Autodesk Inventor part; units mm, degrees
(part 2 of 3)
  line L262 (13.6018, -17.5742) -> (13.2961, -17.2686)
  spline S264 degree 2 poles (13.2961, -17.2686) (13.3171, -17.2092) (13.3852, -17.0328) (13.4219, -16.9716) knots 0 0 0 1 2 2 2
  spline S265 degree 2 poles (13.4219, -16.9716) (13.4708, -16.8808) (13.5599, -16.7498) (13.6454, -16.6642) knots 0 0 0 1 2 2 2
  spline S266 degree 2 poles (12.2779, -18.0318) (12.4455, -17.8641) (12.8263, -17.6895) (13.0306, -17.6947) knots 0 0 0 1 2 2 2
  spline S267 degree 2 poles (13.0306, -17.6947) (13.2332, -17.6982) (13.6612, -17.906) (13.8742, -18.1191) knots 0 0 0 1 2 2 2
  spline S268 degree 2 poles (13.8742, -18.1191) (14.0873, -18.3322) (14.2847, -18.7566) (14.2934, -18.9575) knots 0 0 0 1 2 2 2
  spline S269 degree 2 poles (14.2934, -18.9575) (14.3039, -19.1601) (14.1327, -19.5583) (13.9686, -19.7225) knots 0 0 0 1 2 2 2
  spline S270 degree 2 poles (13.9686, -19.7225) (13.8358, -19.8552) (13.5127, -20.0281) (13.3677, -20.0753) knots 0 0 0 1 2 2 2
  line L263 (13.3677, -20.0753) -> (13.0621, -19.7696)
  line L264 (13.0621, -19.7696) -> (13.0778, -19.7539)
  spline S271 degree 2 poles (13.0778, -19.7539) (13.1319, -19.7487) (13.2856, -19.7207) (13.3835, -19.6893) knots 0 0 0 1 2 2 2
  spline S272 degree 2 poles (13.3835, -19.6893) (13.469, -19.6596) (13.6664, -19.5496) (13.7363, -19.4797) knots 0 0 0 1 2 2 2
  spline S273 degree 2 poles (13.7363, -19.4797) (13.9476, -19.2684) (13.8847, -18.692) (13.593, -18.4003) knots 0 0 0 1 2 2 2
  spline S274 degree 2 poles (13.593, -18.4003) (13.3084, -18.1156) (12.7407, -18.044) (12.5207, -18.2641) knots 0 0 0 1 2 2 2
  spline S275 degree 2 poles (12.5207, -18.2641) (12.3879, -18.3968) (12.2569, -18.7479) (12.2499, -18.926) knots 0 0 0 1 2 2 2
  line L265 (12.2499, -18.926) -> (12.2342, -18.9418)
  line L266 (12.2342, -18.9418) -> (11.9286, -18.6361)
  spline S276 degree 2 poles (11.9286, -18.6361) (11.9495, -18.5767) (12.0176, -18.4003) (12.0543, -18.3392) knots 0 0 0 1 2 2 2
  spline S277 degree 2 poles (12.0543, -18.3392) (12.1032, -18.2484) (12.1923, -18.1174) (12.2779, -18.0318) knots 0 0 0 1 2 2 2
  line L267 (11.312, -19.071) -> (11.5845, -18.7985)
  line L268 (11.5845, -18.7985) -> (13.2018, -20.4159)
  line L269 (13.2018, -20.4159) -> (12.9293, -20.6883)
  line L270 (12.9293, -20.6883) -> (11.312, -19.071)
  line L271 (13.1791, -20.9765) -> (13.4882, -20.6674)
  line L272 (13.4882, -20.6674) -> (13.7712, -20.9503)
  line L273 (13.7712, -20.9503) -> (13.462, -21.2595)
  line L274 (13.462, -21.2595) -> (13.1791, -20.9765)
  spline S278 degree 2 poles (10.3916, -21.6088) (9.9829, -21.2001) (9.9305, -20.3617) (10.2588, -20.0334) knots 0 0 0 1 2 2 2
  spline S279 degree 2 poles (10.2588, -20.0334) (10.5959, -19.6963) (11.4413, -19.7696) (11.836, -20.1644) knots 0 0 0 1 2 2 2
  spline S280 degree 2 poles (11.836, -20.1644) (12.2412, -20.5696) (12.2919, -21.4166) (11.967, -21.7415) knots 0 0 0 1 2 2 2
  spline S281 degree 2 poles (11.967, -21.7415) (11.6386, -22.0699) (10.7985, -22.0157) (10.3916, -21.6088) knots 0 0 0 1 2 2 2
  spline S282 degree 2 poles (10.6728, -21.3276) (10.9872, -21.642) (11.5216, -21.7188) (11.7329, -21.5075) knots 0 0 0 1 2 2 2
  spline S283 degree 2 poles (11.7329, -21.5075) (11.9443, -21.2961) (11.8692, -20.7599) (11.5548, -20.4456) knots 0 0 0 1 2 2 2
  spline S284 degree 2 poles (11.5548, -20.4456) (11.2492, -20.1399) (10.7042, -20.0561) (10.4929, -20.2674) knots 0 0 0 1 2 2 2
  spline S285 degree 2 poles (10.4929, -20.2674) (10.2833, -20.477) (10.3619, -21.0167) (10.6728, -21.3276) knots 0 0 0 1 2 2 2
  line L275 (14.7087, -8.5772) -> (15.9575, -7.3284)
  line L276 (15.9575, -7.3284) -> (18.1127, -9.4837)
  line L277 (18.1127, -9.4837) -> (17.8263, -9.7701)
  line L278 (17.8263, -9.7701) -> (15.926, -7.8699)
  line L279 (15.926, -7.8699) -> (14.9637, -8.8322)
  line L280 (14.9637, -8.8322) -> (14.7087, -8.5772)
  spline S286 degree 2 poles (13.7655, -9.447) (14.1533, -9.0593) (15.0143, -9.068) (15.416, -9.4697) knots 0 0 0 1 2 2 2
  spline S287 degree 2 poles (15.416, -9.4697) (15.8107, -9.8644) (15.8649, -10.7464) (15.5313, -11.08) knots 0 0 0 1 2 2 2
  spline S288 degree 2 poles (15.5313, -11.08) (15.3811, -11.2302) (15.0615, -11.3752) (14.8833, -11.3682) knots 0 0 0 1 2 2 2
  spline S289 degree 2 poles (14.8833, -11.3682) (14.7034, -11.363) (14.3436, -11.1883) (14.1498, -10.9945) knots 0 0 0 1 2 2 2
  line L281 (14.1498, -10.9945) -> (14.0013, -10.846)
  line L282 (14.0013, -10.846) -> (15.1209, -9.7265)
  spline S290 degree 2 poles (15.1209, -9.7265) (14.8397, -9.4453) (14.258, -9.4295) (14.0065, -9.681) knots 0 0 0 1 2 2 2
  spline S291 degree 2 poles (14.0065, -9.681) (13.9175, -9.7701) (13.7847, -9.9832) (13.7463, -10.0845) knots 0 0 0 1 2 2 2
  spline S292 degree 2 poles (13.7463, -10.0845) (13.7079, -10.1928) (13.6677, -10.3552) (13.6625, -10.4163) knots 0 0 0 1 2 2 2
  line L283 (13.6625, -10.4163) -> (13.6468, -10.4321)
  line L284 (13.6468, -10.4321) -> (13.3498, -10.1351)
  spline S293 degree 2 poles (13.3498, -10.1351) (13.3778, -10.0688) (13.4651, -9.8697) (13.5053, -9.7981) knots 0 0 0 1 2 2 2
  spline S294 degree 2 poles (13.5053, -9.7981) (13.5612, -9.6968) (13.6677, -9.5448) (13.7655, -9.447) knots 0 0 0 1 2 2 2
  spline S295 degree 2 poles (14.4746, -10.7884) (14.5881, -10.8949) (14.7942, -11.0102) (14.8921, -11.0207) knots 0 0 0 1 2 2 2
  spline S296 degree 2 poles (14.8921, -11.0207) (15.0003, -11.0346) (15.2134, -10.9508) (15.3235, -10.8408) knots 0 0 0 1 2 2 2
  spline S297 degree 2 poles (15.3235, -10.8408) (15.4317, -10.7325) (15.5191, -10.5159) (15.5191, -10.3901) knots 0 0 0 1 2 2 2
  spline S298 degree 2 poles (15.5191, -10.3901) (15.5156, -10.2644) (15.423, -10.0461) (15.3287, -9.9343) knots 0 0 0 1 2 2 2
  line L285 (15.3287, -9.9343) -> (14.4746, -10.7884)
  spline S299 degree 2 poles (12.4242, -12.479) (12.0155, -12.0703) (11.9631, -11.232) (12.2914, -10.9036) knots 0 0 0 1 2 2 2
  spline S300 degree 2 poles (12.2914, -10.9036) (12.6285, -10.5665) (13.4738, -10.6399) (13.8686, -11.0346) knots 0 0 0 1 2 2 2
  spline S301 degree 2 poles (13.8686, -11.0346) (14.2738, -11.4398) (14.3244, -12.2869) (13.9996, -12.6118) knots 0 0 0 1 2 2 2
  spline S302 degree 2 poles (13.9996, -12.6118) (13.6712, -12.9401) (12.8311, -12.886) (12.4242, -12.479) knots 0 0 0 1 2 2 2
  spline S303 degree 2 poles (12.7054, -12.1978) (13.0197, -12.5122) (13.5542, -12.5891) (13.7655, -12.3777) knots 0 0 0 1 2 2 2
  spline S304 degree 2 poles (13.7655, -12.3777) (13.9769, -12.1664) (13.9017, -11.6302) (13.5874, -11.3158) knots 0 0 0 1 2 2 2
  spline S305 degree 2 poles (13.5874, -11.3158) (13.2817, -11.0102) (12.7368, -10.9263) (12.5255, -11.1377) knots 0 0 0 1 2 2 2
  spline S306 degree 2 poles (12.5255, -11.1377) (12.3159, -11.3473) (12.3945, -11.887) (12.7054, -12.1978) knots 0 0 0 1 2 2 2
  line L286 (10.0663, -13.2196) -> (10.3388, -12.9471)
  line L287 (10.3388, -12.9471) -> (11.2609, -13.8693)
  spline S307 degree 2 poles (11.2609, -13.8693) (11.3727, -13.9811) (11.5858, -14.1522) (11.6749, -14.1784) knots 0 0 0 1 2 2 2
  spline S308 degree 2 poles (11.6749, -14.1784) (11.7692, -14.2064) (11.9473, -14.147) (12.0486, -14.0457) knots 0 0 0 1 2 2 2
  spline S309 degree 2 poles (12.0486, -14.0457) (12.1499, -13.9444) (12.2565, -13.6213) (12.2722, -13.4309) knots 0 0 0 1 2 2 2
  line L288 (12.2722, -13.4309) -> (11.0636, -12.2223)
  line L289 (11.0636, -12.2223) -> (11.336, -11.9498)
  line L290 (11.336, -11.9498) -> (12.9534, -13.5671)
  line L291 (12.9534, -13.5671) -> (12.6809, -13.8396)
  line L292 (12.6809, -13.8396) -> (12.501, -13.6597)
  spline S310 degree 2 poles (12.501, -13.6597) (12.4888, -13.892) (12.3683, -14.2431) (12.2355, -14.3758) knots 0 0 0 1 2 2 2
  spline S311 degree 2 poles (12.2355, -14.3758) (11.998, -14.6133) (11.4146, -14.5679) (11.116, -14.2693) knots 0 0 0 1 2 2 2
  line L293 (11.116, -14.2693) -> (10.0663, -13.2196)
  spline S312 degree 2 poles (8.9537, -14.6745) (8.9625, -14.6168) (8.9869, -14.4177) (9.0131, -14.3391) knots 0 0 0 1 2 2 2
  spline S313 degree 2 poles (9.0131, -14.3391) (9.0463, -14.2291) (9.1406, -14.0544) (9.2629, -13.9322) knots 0 0 0 1 2 2 2
  spline S314 degree 2 poles (9.2629, -13.9322) (9.3624, -13.8326) (9.6174, -13.7278) (9.7537, -13.7278) knots 0 0 0 1 2 2 2
  spline S315 degree 2 poles (9.7537, -13.7278) (9.8846, -13.7296) (10.1589, -13.8466) (10.2671, -13.9549) knots 0 0 0 1 2 2 2
  spline S316 degree 2 poles (10.2671, -13.9549) (10.4348, -14.1226) (10.5309, -14.5016) (10.4453, -14.7234) knots 0 0 0 1 2 2 2
  spline S317 degree 2 poles (10.4453, -14.7234) (10.3719, -14.9225) (10.0488, -15.3399) (9.8462, -15.567) knots 0 0 0 1 2 2 2
  line L294 (9.8462, -15.567) -> (9.8986, -15.6194)
  spline S318 degree 2 poles (9.8986, -15.6194) (9.9929, -15.7137) (10.1676, -15.7731) (10.2532, -15.7538) knots 0 0 0 1 2 2 2
  spline S319 degree 2 poles (10.2532, -15.7538) (10.3388, -15.7346) (10.5099, -15.6054) (10.5903, -15.525) knots 0 0 0 1 2 2 2
  spline S320 degree 2 poles (10.5903, -15.525) (10.6846, -15.4307) (10.8837, -15.1198) (10.957, -14.9382) knots 0 0 0 1 2 2 2
  line L295 (10.957, -14.9382) -> (10.9728, -14.9225)
  line L296 (10.9728, -14.9225) -> (11.2505, -15.2002)
  spline S321 degree 2 poles (11.2505, -15.2002) (11.1963, -15.2962) (10.9675, -15.6298) (10.8295, -15.7678) knots 0 0 0 1 2 2 2
  spline S322 degree 2 poles (10.8295, -15.7678) (10.6619, -15.9355) (10.3807, -16.1119) (10.2217, -16.1346) knots 0 0 0 1 2 2 2
  spline S323 degree 2 poles (10.2217, -16.1346) (10.0663, -16.1573) (9.7676, -16.0333) (9.6157, -15.8813) knots 0 0 0 1 2 2 2
  line L297 (9.6157, -15.8813) -> (8.5101, -14.7758)
  line L298 (8.5101, -14.7758) -> (8.7826, -14.5033)
  line L299 (8.7826, -14.5033) -> (8.9537, -14.6745)
  line L300 (9.1808, -14.9015) -> (9.6297, -15.3504)
  spline S324 degree 2 poles (9.6297, -15.3504) (9.7187, -15.2439) (9.9842, -14.919) (10.0488, -14.7985) knots 0 0 0 1 2 2 2
  spline S325 degree 2 poles (10.0488, -14.7985) (10.1239, -14.657) (10.1274, -14.3776) (10.0052, -14.2553) knots 0 0 0 1 2 2 2
  spline S326 degree 2 poles (10.0052, -14.2553) (9.8654, -14.1156) (9.5668, -14.1313) (9.4166, -14.2815) knots 0 0 0 1 2 2 2
  spline S327 degree 2 poles (9.4166, -14.2815) (9.2891, -14.409) (9.1895, -14.7286) (9.1808, -14.9015) knots 0 0 0 1 2 2 2
  line L301 (8.5957, -17.3415) -> (8.6097, -17.3275)
  spline S328 degree 2 poles (8.6097, -17.3275) (8.6498, -17.3048) (8.7214, -17.2402) (8.7686, -17.193) knots 0 0 0 1 2 2 2
  spline S329 degree 2 poles (8.7686, -17.193) (8.8786, -17.083) (8.9991, -16.7703) (9.0026, -16.5782) knots 0 0 0 1 2 2 2
  line L302 (9.0026, -16.5782) -> (7.8551, -15.4307)
  line L303 (7.8551, -15.4307) -> (8.1276, -15.1583)
  line L304 (8.1276, -15.1583) -> (9.7449, -16.7756)
  line L305 (9.7449, -16.7756) -> (9.4725, -17.0481)
  line L306 (9.4725, -17.0481) -> (9.2314, -16.807)
  spline S330 degree 2 poles (9.2314, -16.807) (9.2157, -17.0882) (9.1022, -17.4183) (8.9974, -17.5231) knots 0 0 0 1 2 2 2
  spline S331 degree 2 poles (8.9974, -17.5231) (8.9555, -17.565) (8.9101, -17.6035) (8.8786, -17.6244) knots 0 0 0 1 2 2 2
  line L307 (8.8786, -17.6244) -> (8.5957, -17.3415)
  line L308 (5.8152, -17.4707) -> (6.0876, -17.1983)
  line L309 (6.0876, -17.1983) -> (6.2518, -17.3624)
  spline S332 degree 2 poles (6.2518, -17.3624) (6.2623, -17.2472) (6.285, -17.0847) (6.3182, -16.9922) knots 0 0 0 1 2 2 2
  spline S333 degree 2 poles (6.3182, -16.9922) (6.3479, -16.9066) (6.4422, -16.7529) (6.5243, -16.6708) knots 0 0 0 1 2 2 2
  spline S334 degree 2 poles (6.5243, -16.6708) (6.657, -16.5381) (6.9906, -16.4245) (7.1757, -16.4525) knots 0 0 0 1 2 2 2
  spline S335 degree 2 poles (7.1757, -16.4525) (7.3609, -16.4804) (7.7626, -16.7075) (7.9669, -16.9118) knots 0 0 0 1 2 2 2
  spline S336 degree 2 poles (7.9669, -16.9118) (8.18, -17.1249) (8.3809, -17.5458) (8.4018, -17.7589) knots 0 0 0 1 2 2 2
  spline S337 degree 2 poles (8.4018, -17.7589) (8.4175, -17.9528) (8.2883, -18.323) (8.1503, -18.461) knots 0 0 0 1 2 2 2
  spline S338 degree 2 poles (8.1503, -18.461) (8.0298, -18.5815) (7.7958, -18.7073) (7.6403, -18.751) knots 0 0 0 1 2 2 2
  line L310 (7.6403, -18.751) -> (8.3389, -19.4496)
  line L311 (8.3389, -19.4496) -> (8.0665, -19.722)
  line L312 (8.0665, -19.722) -> (5.8152, -17.4707)
  line L313 (6.4806, -17.5912) -> (7.415, -18.5256)
  spline S339 degree 2 poles (7.415, -18.5256) (7.5652, -18.4732) (7.7626, -18.3492) (7.8551, -18.2567) knots 0 0 0 1 2 2 2
  spline S340 degree 2 poles (7.8551, -18.2567) (8.0647, -18.0471) (7.9879, -17.4952) (7.691, -17.1983) knots 0 0 0 1 2 2 2
  spline S341 degree 2 poles (7.691, -17.1983) (7.4045, -16.9118) (6.9207, -16.7913) (6.7199, -16.9922) knots 0 0 0 1 2 2 2
  spline S342 degree 2 poles (6.7199, -16.9922) (6.6133, -17.0987) (6.4946, -17.4131) (6.4806, -17.5912) knots 0 0 0 1 2 2 2
  spline S343 degree 2 poles (4.9, -20.0032) (4.4913, -19.5945) (4.4389, -18.7562) (4.7672, -18.4278) knots 0 0 0 1 2 2 2
  spline S344 degree 2 poles (4.7672, -18.4278) (5.1043, -18.0908) (5.9496, -18.1641) (6.3444, -18.5588) knots 0 0 0 1 2 2 2
  spline S345 degree 2 poles (6.3444, -18.5588) (6.7496, -18.964) (6.8002, -19.8111) (6.4754, -20.136) knots 0 0 0 1 2 2 2
  spline S346 degree 2 poles (6.4754, -20.136) (6.147, -20.4643) (5.3069, -20.4102) (4.9, -20.0032) knots 0 0 0 1 2 2 2
  spline S347 degree 2 poles (5.1811, -19.722) (5.4955, -20.0364) (6.03, -20.1133) (6.2413, -19.9019) knots 0 0 0 1 2 2 2
  spline S348 degree 2 poles (6.2413, -19.9019) (6.4526, -19.6906) (6.3775, -19.1544) (6.0632, -18.84) knots 0 0 0 1 2 2 2
  spline S349 degree 2 poles (6.0632, -18.84) (5.7575, -18.5344) (5.2126, -18.4505) (5.0013, -18.6619) knots 0 0 0 1 2 2 2
  spline S350 degree 2 poles (5.0013, -18.6619) (4.7917, -18.8715) (4.8703, -19.4112) (5.1811, -19.722) knots 0 0 0 1 2 2 2
  line L314 (-17.3745, -18.836) -> (-14.477, -17.4231)
  line L315 (-14.477, -17.4231) -> (-14.1679, -17.7322)
  line L316 (-14.1679, -17.7322) -> (-15.5808, -20.6297)
  line L317 (-15.5808, -20.6297) -> (-15.8882, -20.3224)
  line L318 (-15.8882, -20.3224) -> (-14.6953, -17.9348)
  line L319 (-14.6953, -17.9348) -> (-17.0829, -19.1277)
  line L320 (-17.0829, -19.1277) -> (-17.3745, -18.836)
  line L321 (-15.6821, -16.2179) -> (-15.4097, -16.4904)
  line L322 (-15.4097, -16.4904) -> (-17.027, -18.1077)
  line L323 (-17.027, -18.1077) -> (-17.2994, -17.8352)
  line L324 (-17.2994, -17.8352) -> (-15.6821, -16.2179)
  line L325 (-17.5876, -18.085) -> (-17.2785, -18.3941)
  line L326 (-17.2785, -18.3941) -> (-17.5614, -18.6771)
  line L327 (-17.5614, -18.6771) -> (-17.8706, -18.3679)
  line L328 (-17.8706, -18.3679) -> (-17.5876, -18.085)
  spline S351 degree 2 poles (-16.5397, -15.2975) (-16.3179, -15.5193) (-16.3214, -16.0223) (-16.5956, -16.2965) knots 0 0 0 1 2 2 2
  line L329 (-16.5956, -16.2965) -> (-17.4916, -17.1925)
  line L330 (-17.4916, -17.1925) -> (-17.3082, -17.3759)
  line L331 (-17.3082, -17.3759) -> (-17.5335, -17.6012)
  line L332 (-17.5335, -17.6012) -> (-17.7169, -17.4178)
  line L333 (-17.7169, -17.4178) -> (-18.1815, -17.8824)
  line L334 (-18.1815, -17.8824) -> (-18.4539, -17.6099)
  line L335 (-18.4539, -17.6099) -> (-17.9893, -17.1454)
  line L336 (-17.9893, -17.1454) -> (-18.4906, -16.6441)
  line L337 (-18.4906, -16.6441) -> (-18.2653, -16.4188)
  line L338 (-18.2653, -16.4188) -> (-17.764, -16.92)
  line L339 (-17.764, -16.92) -> (-16.9938, -16.1498)
  spline S352 degree 2 poles (-16.9938, -16.1498) (-16.8715, -16.0275) (-16.7458, -15.8843) (-16.7178, -15.797) knots 0 0 0 1 2 2 2
  spline S353 degree 2 poles (-16.7178, -15.797) (-16.6916, -15.7219) (-16.751, -15.5612) (-16.8453, -15.4669) knots 0 0 0 1 2 2 2
  spline S354 degree 2 poles (-16.8453, -15.4669) (-16.9117, -15.4005) (-17.0759, -15.3167) (-17.1161, -15.301) knots 0 0 0 1 2 2 2
  line L340 (-17.1161, -15.301) -> (-17.1318, -15.2853)
  line L341 (-17.1318, -15.2853) -> (-16.8873, -15.0407)
  spline S355 degree 2 poles (-16.8873, -15.0407) (-16.7894, -15.0966) (-16.6078, -15.2294) (-16.5397, -15.2975) knots 0 0 0 1 2 2 2
  spline S356 degree 2 poles (-17.5317, -14.3054) (-17.3099, -14.5272) (-17.3134, -15.0303) (-17.5876, -15.3045) knots 0 0 0 1 2 2 2
  line L342 (-17.5876, -15.3045) -> (-18.4836, -16.2005)
  line L343 (-18.4836, -16.2005) -> (-18.3002, -16.3838)
  line L344 (-18.3002, -16.3838) -> (-18.5255, -16.6092)
  line L345 (-18.5255, -16.6092) -> (-18.7089, -16.4258)
  line L346 (-18.7089, -16.4258) -> (-19.1735, -16.8904)
  line L347 (-19.1735, -16.8904) -> (-19.446, -16.6179)
  line L348 (-19.446, -16.6179) -> (-18.9814, -16.1533)
  line L349 (-18.9814, -16.1533) -> (-19.4827, -15.652)
  line L350 (-19.4827, -15.652) -> (-19.2573, -15.4267)
  line L351 (-19.2573, -15.4267) -> (-18.7561, -15.928)
  line L352 (-18.7561, -15.928) -> (-17.9858, -15.1578)
  spline S357 degree 2 poles (-17.9858, -15.1578) (-17.8636, -15.0355) (-17.7378, -14.8923) (-17.7099, -14.805) knots 0 0 0 1 2 2 2
  spline S358 degree 2 poles (-17.7099, -14.805) (-17.6837, -14.7299) (-17.7431, -14.5692) (-17.8374, -14.4749) knots 0 0 0 1 2 2 2
  spline S359 degree 2 poles (-17.8374, -14.4749) (-17.9038, -14.4085) (-18.0679, -14.3246) (-18.1081, -14.3089) knots 0 0 0 1 2 2 2
  line L353 (-18.1081, -14.3089) -> (-18.1238, -14.2932)
  line L354 (-18.1238, -14.2932) -> (-17.8793, -14.0487)
  spline S360 degree 2 poles (-17.8793, -14.0487) (-17.7815, -14.1046) (-17.5999, -14.2373) (-17.5317, -14.3054) knots 0 0 0 1 2 2 2
  line L355 (-18.3439, -13.5562) -> (-18.0714, -13.8286)
  line L356 (-18.0714, -13.8286) -> (-19.6887, -15.4459)
  line L357 (-19.6887, -15.4459) -> (-19.9612, -15.1735)
  line L358 (-19.9612, -15.1735) -> (-18.3439, -13.5562)
  line L359 (-20.2494, -15.4232) -> (-19.9403, -15.7324)
  line L360 (-19.9403, -15.7324) -> (-20.2232, -16.0153)
  line L361 (-20.2232, -16.0153) -> (-20.5323, -15.7062)
  line L362 (-20.5323, -15.7062) -> (-20.2494, -15.4232)
  spline S361 degree 2 poles (-8.1645, -16.5546) (-7.9357, -16.7834) (-7.6964, -17.3021) (-7.7016, -17.5798) knots 0 0 0 1 2 2 2
  spline S362 degree 2 poles (-7.7016, -17.5798) (-7.7086, -17.8593) (-7.9863, -18.4269) (-8.2605, -18.7011) knots 0 0 0 1 2 2 2
  spline S363 degree 2 poles (-8.2605, -18.7011) (-8.5208, -18.9613) (-9.0797, -19.2268) (-9.3626, -19.2373) knots 0 0 0 1 2 2 2
  spline S364 degree 2 poles (-9.3626, -19.2373) (-9.6351, -19.2478) (-10.173, -19.0172) (-10.4018, -18.7884) knots 0 0 0 1 2 2 2
  spline S365 degree 2 poles (-10.4018, -18.7884) (-10.5119, -18.6784) (-10.6795, -18.4479) (-10.7424, -18.3291) knots 0 0 0 1 2 2 2
  spline S366 degree 2 poles (-10.7424, -18.3291) (-10.7948, -18.2348) (-10.8961, -17.9798) (-10.9223, -17.8977) knots 0 0 0 1 2 2 2
  line L363 (-10.9223, -17.8977) -> (-10.5765, -17.5519)
  line L364 (-10.5765, -17.5519) -> (-10.552, -17.5763)
  spline S367 degree 2 poles (-10.552, -17.5763) (-10.545, -17.6776) (-10.5171, -17.8767) (-10.4612, -18.0304) knots 0 0 0 1 2 2 2
  spline S368 degree 2 poles (-10.4612, -18.0304) (-10.4175, -18.1614) (-10.2499, -18.4444) (-10.1206, -18.5736) knots 0 0 0 1 2 2 2
  spline S369 degree 2 poles (-10.1206, -18.5736) (-9.8097, -18.8845) (-8.9574, -18.8007) (-8.5679, -18.4112) knots 0 0 0 1 2 2 2
  spline S370 degree 2 poles (-8.5679, -18.4112) (-8.3514, -18.1946) (-8.1278, -17.7684) (-8.1121, -17.5606) knots 0 0 0 1 2 2 2
  spline S371 degree 2 poles (-8.1121, -17.5606) (-8.0929, -17.3563) (-8.2378, -16.9772) (-8.402, -16.8131) knots 0 0 0 1 2 2 2
  spline S372 degree 2 poles (-8.402, -16.8131) (-8.5225, -16.6926) (-8.7985, -16.4865) (-8.9155, -16.4393) knots 0 0 0 1 2 2 2
  line L365 (-8.9155, -16.4393) -> (-9.4727, -16.9965)
  line L366 (-9.4727, -16.9965) -> (-8.9731, -17.496)
  line L367 (-8.9731, -17.496) -> (-9.2246, -17.7475)
  line L368 (-9.2246, -17.7475) -> (-10.0071, -16.965)
  line L369 (-10.0071, -16.965) -> (-9.0657, -16.0236)
  spline S373 degree 2 poles (-9.0657, -16.0236) (-8.9871, -16.0533) (-8.7269, -16.1633) (-8.6256, -16.2192) knots 0 0 0 1 2 2 2
  spline S374 degree 2 poles (-8.6256, -16.2192) (-8.4876, -16.2943) (-8.285, -16.4341) (-8.1645, -16.5546) knots 0 0 0 1 2 2 2
  spline S375 degree 2 poles (-10.3337, -14.8115) (-10.2761, -14.8202) (-10.077, -14.8447) (-9.9984, -14.8709) knots 0 0 0 1 2 2 2
  spline S376 degree 2 poles (-9.9984, -14.8709) (-9.8883, -14.9041) (-9.7137, -14.9984) (-9.5914, -15.1206) knots 0 0 0 1 2 2 2
  spline S377 degree 2 poles (-9.5914, -15.1206) (-9.4919, -15.2202) (-9.3871, -15.4752) (-9.3871, -15.6114) knots 0 0 0 1 2 2 2
  spline S378 degree 2 poles (-9.3871, -15.6114) (-9.3888, -15.7424) (-9.5058, -16.0166) (-9.6141, -16.1249) knots 0 0 0 1 2 2 2
  spline S379 degree 2 poles (-9.6141, -16.1249) (-9.7818, -16.2926) (-10.1608, -16.3887) (-10.3826, -16.3031) knots 0 0 0 1 2 2 2
  spline S380 degree 2 poles (-10.3826, -16.3031) (-10.5817, -16.2297) (-10.9992, -15.9066) (-11.2262, -15.704) knots 0 0 0 1 2 2 2
  line L370 (-11.2262, -15.704) -> (-11.2786, -15.7564)
  spline S381 degree 2 poles (-11.2786, -15.7564) (-11.3729, -15.8507) (-11.4323, -16.0254) (-11.4131, -16.111) knots 0 0 0 1 2 2 2
  spline S382 degree 2 poles (-11.4131, -16.111) (-11.3939, -16.1965) (-11.2646, -16.3677) (-11.1843, -16.448) knots 0 0 0 1 2 2 2
  spline S383 degree 2 poles (-11.1843, -16.448) (-11.09, -16.5424) (-10.7791, -16.7415) (-10.5974, -16.8148) knots 0 0 0 1 2 2 2
  line L371 (-10.5974, -16.8148) -> (-10.5817, -16.8305)
  line L372 (-10.5817, -16.8305) -> (-10.8594, -17.1082)
  spline S384 degree 2 poles (-10.8594, -17.1082) (-10.9555, -17.0541) (-11.2891, -16.8253) (-11.4271, -16.6873) knots 0 0 0 1 2 2 2
  spline S385 degree 2 poles (-11.4271, -16.6873) (-11.5947, -16.5196) (-11.7711, -16.2384) (-11.7938, -16.0795) knots 0 0 0 1 2 2 2
  spline S386 degree 2 poles (-11.7938, -16.0795) (-11.8165, -15.9241) (-11.6925, -15.6254) (-11.5406, -15.4735) knots 0 0 0 1 2 2 2
  line L373 (-11.5406, -15.4735) -> (-10.435, -14.3679)
  line L374 (-10.435, -14.3679) -> (-10.1625, -14.6403)
  line L375 (-10.1625, -14.6403) -> (-10.3337, -14.8115)
  line L376 (-10.5608, -15.0386) -> (-11.0096, -15.4874)
  spline S387 degree 2 poles (-11.0096, -15.4874) (-10.9031, -15.5765) (-10.5782, -15.842) (-10.4577, -15.9066) knots 0 0 0 1 2 2 2
  spline S388 degree 2 poles (-10.4577, -15.9066) (-10.3162, -15.9817) (-10.0368, -15.9852) (-9.9145, -15.8629) knots 0 0 0 1 2 2 2
  spline S389 degree 2 poles (-9.9145, -15.8629) (-9.7748, -15.7232) (-9.7905, -15.4246) (-9.9407, -15.2743) knots 0 0 0 1 2 2 2
  spline S390 degree 2 poles (-9.9407, -15.2743) (-10.0682, -15.1468) (-10.3879, -15.0473) (-10.5608, -15.0386) knots 0 0 0 1 2 2 2
  spline S391 degree 2 poles (-13.0077, -13.4649) (-12.6112, -13.0684) (-11.7432, -12.9689) (-11.4533, -13.2588) knots 0 0 0 1 2 2 2
  spline S392 degree 2 poles (-11.4533, -13.2588) (-11.3223, -13.3898) (-11.2, -13.6413) (-11.1651, -13.788) knots 0 0 0 1 2 2 2
  line L377 (-11.1651, -13.788) -> (-11.0725, -13.7304)
  line L378 (-11.0725, -13.7304) -> (-10.8175, -13.9854)
  line L379 (-10.8175, -13.9854) -> (-13.0688, -16.2367)
  line L380 (-13.0688, -16.2367) -> (-13.3413, -15.9642)
  line L381 (-13.3413, -15.9642) -> (-12.5379, -15.1608)
  spline S393 degree 2 poles (-12.5379, -15.1608) (-12.7335, -15.1503) (-13.095, -15.0333) (-13.247, -14.8814) knots 0 0 0 1 2 2 2
  spline S394 degree 2 poles (-13.247, -14.8814) (-13.5212, -14.6072) (-13.3972, -13.8544) (-13.0077, -13.4649) knots 0 0 0 1 2 2 2
  spline S395 degree 2 poles (-12.7055, -13.7251) (-12.9955, -14.0151) (-13.1195, -14.4919) (-12.9239, -14.6875) knots 0 0 0 1 2 2 2
  spline S396 degree 2 poles (-12.9239, -14.6875) (-12.8138, -14.7975) (-12.482, -14.9198) (-12.3091, -14.932) knots 0 0 0 1 2 2 2
  line L382 (-12.3091, -14.932) -> (-11.3816, -14.0046)
  spline S397 degree 2 poles (-11.3816, -14.0046) (-11.434, -13.8509) (-11.5511, -13.65) (-11.6454, -13.5557) knots 0 0 0 1 2 2 2
  spline S398 degree 2 poles (-11.6454, -13.5557) (-11.8532, -13.3479) (-12.3859, -13.4055) (-12.7055, -13.7251) knots 0 0 0 1 2 2 2
  line L383 (-14.639, -12.8152) -> (-14.625, -12.8292)
  spline S399 degree 2 poles (-14.625, -12.8292) (-14.6023, -12.8693) (-14.5377, -12.9409) (-14.4905, -12.9881) knots 0 0 0 1 2 2 2
  spline S400 degree 2 poles (-14.4905, -12.9881) (-14.3805, -13.0981) (-14.0679, -13.2186) (-13.8757, -13.2221) knots 0 0 0 1 2 2 2
  line L384 (-13.8757, -13.2221) -> (-12.7283, -12.0746)
  line L385 (-12.7283, -12.0746) -> (-12.4558, -12.3471)
  line L386 (-12.4558, -12.3471) -> (-14.0731, -13.9644)
  line L387 (-14.0731, -13.9644) -> (-14.3456, -13.692)
  line L388 (-14.3456, -13.692) -> (-14.1045, -13.4509)
  spline S401 degree 2 poles (-14.1045, -13.4509) (-14.3857, -13.4352) (-14.7158, -13.3217) (-14.8206, -13.2169) knots 0 0 0 1 2 2 2
  spline S402 degree 2 poles (-14.8206, -13.2169) (-14.8626, -13.175) (-14.901, -13.1296) (-14.9219, -13.0981) knots 0 0 0 1 2 2 2
  line L389 (-14.9219, -13.0981) -> (-14.639, -12.8152)
  line L390 (-13.8024, -11.0005) -> (-13.5299, -11.273)
  line L391 (-13.5299, -11.273) -> (-15.1472, -12.8903)
  line L392 (-15.1472, -12.8903) -> (-15.4197, -12.6178)
  line L393 (-15.4197, -12.6178) -> (-13.8024, -11.0005)
  line L394 (-15.7079, -12.8676) -> (-15.3987, -13.1767)
  line L395 (-15.3987, -13.1767) -> (-15.6817, -13.4597)
  line L396 (-15.6817, -13.4597) -> (-15.9908, -13.1505)
  line L397 (-15.9908, -13.1505) -> (-15.7079, -12.8676)
  spline S403 degree 2 poles (-14.8678, -9.8617) (-14.4801, -10.2495) (-14.4888, -11.1105) (-14.8905, -11.5122) knots 0 0 0 1 2 2 2
  spline S404 degree 2 poles (-14.8905, -11.5122) (-15.2852, -11.907) (-16.1672, -11.9611) (-16.5008, -11.6275) knots 0 0 0 1 2 2 2
  spline S405 degree 2 poles (-16.5008, -11.6275) (-16.651, -11.4773) (-16.796, -11.1577) (-16.789, -10.9795) knots 0 0 0 1 2 2 2
  spline S406 degree 2 poles (-16.789, -10.9795) (-16.7838, -10.7996) (-16.6091, -10.4399) (-16.4152, -10.246) knots 0 0 0 1 2 2 2
  line L398 (-16.4152, -10.246) -> (-16.2668, -10.0975)
  line L399 (-16.2668, -10.0975) -> (-15.1472, -11.2171)
  spline S407 degree 2 poles (-15.1472, -11.2171) (-14.866, -10.9359) (-14.8503, -10.3543) (-15.1018, -10.1028) knots 0 0 0 1 2 2 2
  spline S408 degree 2 poles (-15.1018, -10.1028) (-15.1909, -10.0137) (-15.404, -9.881) (-15.5053, -9.8425) knots 0 0 0 1 2 2 2
  spline S409 degree 2 poles (-15.5053, -9.8425) (-15.6136, -9.8041) (-15.776, -9.7639) (-15.8371, -9.7587) knots 0 0 0 1 2 2 2
  line L400 (-15.8371, -9.7587) -> (-15.8529, -9.743)
  line L401 (-15.8529, -9.743) -> (-15.5559, -9.4461)
  spline S410 degree 2 poles (-15.5559, -9.4461) (-15.4896, -9.474) (-15.2905, -9.5613) (-15.2189, -9.6015) knots 0 0 0 1 2 2 2
  spline S411 degree 2 poles (-15.2189, -9.6015) (-15.1176, -9.6574) (-14.9656, -9.7639) (-14.8678, -9.8617) knots 0 0 0 1 2 2 2
  spline S412 degree 2 poles (-16.2092, -10.5708) (-16.3157, -10.6844) (-16.431, -10.8905) (-16.4414, -10.9883) knots 0 0 0 1 2 2 2
  spline S413 degree 2 poles (-16.4414, -10.9883) (-16.4554, -11.0966) (-16.3716, -11.3096) (-16.2616, -11.4197) knots 0 0 0 1 2 2 2
  spline S414 degree 2 poles (-16.2616, -11.4197) (-16.1533, -11.528) (-15.9367, -11.6153) (-15.8109, -11.6153) knots 0 0 0 1 2 2 2
  spline S415 degree 2 poles (-15.8109, -11.6153) (-15.6852, -11.6118) (-15.4669, -11.5192) (-15.3551, -11.4249) knots 0 0 0 1 2 2 2
  line L402 (-15.3551, -11.4249) -> (-16.2092, -10.5708)
  line L403 (-16.0397, -8.7632) -> (-15.7673, -9.0356)
  line L404 (-15.7673, -9.0356) -> (-18.0186, -11.2869)
  line L405 (-18.0186, -11.2869) -> (-18.2911, -11.0145)
  line L406 (-18.2911, -11.0145) -> (-16.0397, -8.7632)
  spline S416 degree 2 poles (-17.1051, -7.6244) (-16.7174, -8.0121) (-16.7261, -8.8732) (-17.1278, -9.2749) knots 0 0 0 1 2 2 2
  spline S417 degree 2 poles (-17.1278, -9.2749) (-17.5226, -9.6696) (-18.4046, -9.7238) (-18.7382, -9.3902) knots 0 0 0 1 2 2 2
  spline S418 degree 2 poles (-18.7382, -9.3902) (-18.8884, -9.24) (-19.0334, -8.9203) (-19.0264, -8.7422) knots 0 0 0 1 2 2 2
  spline S419 degree 2 poles (-19.0264, -8.7422) (-19.0211, -8.5623) (-18.8465, -8.2025) (-18.6526, -8.0086) knots 0 0 0 1 2 2 2
  line L407 (-18.6526, -8.0086) -> (-18.5041, -7.8602)
  line L408 (-18.5041, -7.8602) -> (-17.3846, -8.9797)
  spline S420 degree 2 poles (-17.3846, -8.9797) (-17.1034, -8.6985) (-17.0877, -8.1169) (-17.3392, -7.8654) knots 0 0 0 1 2 2 2
  spline S421 degree 2 poles (-17.3392, -7.8654) (-17.4283, -7.7763) (-17.6413, -7.6436) (-17.7426, -7.6052) knots 0 0 0 1 2 2 2
  spline S422 degree 2 poles (-17.7426, -7.6052) (-17.8509, -7.5668) (-18.0134, -7.5266) (-18.0745, -7.5213) knots 0 0 0 1 2 2 2
  line L409 (-18.0745, -7.5213) -> (-18.0902, -7.5056)
  line L410 (-18.0902, -7.5056) -> (-17.7933, -7.2087)
  spline S423 degree 2 poles (-17.7933, -7.2087) (-17.7269, -7.2367) (-17.5278, -7.324) (-17.4562, -7.3642) knots 0 0 0 1 2 2 2
  spline S424 degree 2 poles (-17.4562, -7.3642) (-17.3549, -7.42) (-17.203, -7.5266) (-17.1051, -7.6244) knots 0 0 0 1 2 2 2
  spline S425 degree 2 poles (-18.4465, -8.3335) (-18.553, -8.447) (-18.6683, -8.6531) (-18.6788, -8.7509) knots 0 0 0 1 2 2 2
  spline S426 degree 2 poles (-18.6788, -8.7509) (-18.6928, -8.8592) (-18.6089, -9.0723) (-18.4989, -9.1823) knots 0 0 0 1 2 2 2
  spline S427 degree 2 poles (-18.4989, -9.1823) (-18.3906, -9.2906) (-18.174, -9.3779) (-18.0483, -9.3779) knots 0 0 0 1 2 2 2
  spline S428 degree 2 poles (-18.0483, -9.3779) (-17.9225, -9.3744) (-17.7042, -9.2819) (-17.5924, -9.1876) knots 0 0 0 1 2 2 2
  line L411 (-17.5924, -9.1876) -> (-18.4465, -8.3335)
  dimension "d28" = 45
  dimension "d29" = 45
  dimension "d30" = 135
  dimension "d31" = 135
  constraints: 16 end point, 4 equal length, 4 horizontal, 8 other
  measures "d28" angle of L16 L17
  measures "d29" angle of L19 L18
  measures "d30" angle of L21 L20
  measures "d31" angle of L22 L23
extrude "Estrusione2" cut sketch "Schizzo4" against normal blind 1
sketch "Schizzo5" plane through (0, 10, 0) normal (0, 1, 0) x (1, 0, 0)
  line L0 (-18.4465, -8.3335) -> (-17.5924, -9.1876) projected
  line L1 (-17.7933, -7.2087) -> (-18.0902, -7.5056) projected
  line L2 (-18.0902, -7.5056) -> (-18.0745, -7.5213) projected
  line L3 (-17.3846, -8.9797) -> (-18.5041, -7.8602) projected
  line L4 (-18.5041, -7.8602) -> (-18.6526, -8.0086) projected
  line L5 (-15.7079, -12.8676) -> (-15.9908, -13.1505) projected
  line L6 (-15.9908, -13.1505) -> (-15.6817, -13.4597) projected
  line L7 (-15.6817, -13.4597) -> (-15.3987, -13.1767) projected
  line L8 (-15.3987, -13.1767) -> (-15.7079, -12.8676) projected
  line L9 (-14.639, -12.8152) -> (-14.9219, -13.0981) projected
  line L10 (-14.1045, -13.4509) -> (-14.3456, -13.692) projected
  line L11 (-14.3456, -13.692) -> (-14.0731, -13.9644) projected
  line L12 (-14.0731, -13.9644) -> (-12.4558, -12.3471) projected
  line L13 (-12.4558, -12.3471) -> (-12.7283, -12.0746) projected
  line L14 (-12.7283, -12.0746) -> (-13.8757, -13.2221) projected
  line L15 (-14.625, -12.8292) -> (-14.639, -12.8152) projected
  line L16 (-11.3816, -14.0046) -> (-12.3091, -14.932) projected
  line L17 (-12.5379, -15.1608) -> (-13.3413, -15.9642) projected
  line L18 (-13.3413, -15.9642) -> (-13.0688, -16.2367) projected
  line L19 (-13.0688, -16.2367) -> (-10.8175, -13.9854) projected
  line L20 (-10.8175, -13.9854) -> (-11.0725, -13.7304) projected
  line L21 (-11.0725, -13.7304) -> (-11.1651, -13.788) projected
  line L22 (-11.0096, -15.4874) -> (-10.5608, -15.0386) projected
  line L23 (-10.3337, -14.8115) -> (-10.1625, -14.6403) projected
  line L24 (-10.1625, -14.6403) -> (-10.435, -14.3679) projected
  line L25 (-10.435, -14.3679) -> (-11.5406, -15.4735) projected
  line L26 (-10.8594, -17.1082) -> (-10.5817, -16.8305) projected
  line L27 (-10.5817, -16.8305) -> (-10.5974, -16.8148) projected
  line L28 (-11.2786, -15.7564) -> (-11.2262, -15.704) projected
  line L29 (-20.2494, -15.4232) -> (-20.5323, -15.7062) projected
  line L30 (-20.5323, -15.7062) -> (-20.2232, -16.0153) projected
  line L31 (-20.2232, -16.0153) -> (-19.9403, -15.7324) projected
  line L32 (-19.9403, -15.7324) -> (-20.2494, -15.4232) projected
  line L33 (-17.8793, -14.0487) -> (-18.1238, -14.2932) projected
  line L34 (-18.1238, -14.2932) -> (-18.1081, -14.3089) projected
  line L35 (-17.9858, -15.1578) -> (-18.7561, -15.928) projected
  line L36 (-18.7561, -15.928) -> (-19.2573, -15.4267) projected
  line L37 (-19.2573, -15.4267) -> (-19.4827, -15.652) projected
  line L38 (-19.4827, -15.652) -> (-18.9814, -16.1533) projected
  line L39 (-18.9814, -16.1533) -> (-19.446, -16.6179) projected
  line L40 (-19.446, -16.6179) -> (-19.1735, -16.8904) projected
  line L41 (-19.1735, -16.8904) -> (-18.7089, -16.4258) projected
  line L42 (-18.7089, -16.4258) -> (-18.5255, -16.6092) projected
  line L43 (-18.5255, -16.6092) -> (-18.3002, -16.3838) projected
  line L44 (-18.3002, -16.3838) -> (-18.4836, -16.2005) projected
  line L45 (-18.4836, -16.2005) -> (-17.5876, -15.3045) projected
  line L46 (-17.5876, -18.085) -> (-17.8706, -18.3679) projected
  line L47 (-17.8706, -18.3679) -> (-17.5614, -18.6771) projected
  line L48 (-17.5614, -18.6771) -> (-17.2785, -18.3941) projected
  line L49 (-17.2785, -18.3941) -> (-17.5876, -18.085) projected
  line L50 (-17.3745, -18.836) -> (-17.0829, -19.1277) projected
  line L51 (-17.0829, -19.1277) -> (-14.6953, -17.9348) projected
  line L52 (-14.6953, -17.9348) -> (-15.8882, -20.3224) projected
  line L53 (-15.8882, -20.3224) -> (-15.5808, -20.6297) projected
  line L54 (-15.5808, -20.6297) -> (-14.1679, -17.7322) projected
  line L55 (-14.1679, -17.7322) -> (-14.477, -17.4231) projected
  line L56 (-14.477, -17.4231) -> (-17.3745, -18.836) projected
  line L57 (7.415, -18.5256) -> (6.4806, -17.5912) projected
  line L58 (5.8152, -17.4707) -> (8.0665, -19.722) projected
  line L59 (8.0665, -19.722) -> (8.3389, -19.4496) projected
  line L60 (8.3389, -19.4496) -> (7.6403, -18.751) projected
  line L61 (6.2518, -17.3624) -> (6.0876, -17.1983) projected
  line L62 (6.0876, -17.1983) -> (5.8152, -17.4707) projected
  line L63 (10.0663, -13.2196) -> (11.116, -14.2693) projected
  line L64 (12.501, -13.6597) -> (12.6809, -13.8396) projected
  line L65 (12.6809, -13.8396) -> (12.9534, -13.5671) projected
  line L66 (12.9534, -13.5671) -> (11.336, -11.9498) projected
  line L67 (11.336, -11.9498) -> (11.0636, -12.2223) projected
  line L68 (11.0636, -12.2223) -> (12.2722, -13.4309) projected
  line L69 (11.2609, -13.8693) -> (10.3388, -12.9471) projected
  line L70 (10.3388, -12.9471) -> (10.0663, -13.2196) projected
  line L71 (14.4746, -10.7884) -> (15.3287, -9.9343) projected
  line L72 (13.3498, -10.1351) -> (13.6468, -10.4321) projected
  line L73 (13.6468, -10.4321) -> (13.6625, -10.4163) projected
  line L74 (15.1209, -9.7265) -> (14.0013, -10.846) projected
  line L75 (14.0013, -10.846) -> (14.1498, -10.9945) projected
  line L76 (13.1791, -20.9765) -> (13.462, -21.2595) projected
  line L77 (13.462, -21.2595) -> (13.7712, -20.9503) projected
  line L78 (13.7712, -20.9503) -> (13.4882, -20.6674) projected
  line L79 (13.4882, -20.6674) -> (13.1791, -20.9765) projected
  line L80 (11.9286, -18.6361) -> (12.2342, -18.9418) projected
  line L81 (12.2342, -18.9418) -> (12.2499, -18.926) projected
  line L82 (13.0778, -19.7539) -> (13.0621, -19.7696) projected
  line L83 (13.0621, -19.7696) -> (13.3677, -20.0753) projected
  line L84 (18.0206, -15.7857) -> (17.9996, -15.8067) projected
  line L85 (17.9996, -15.8067) -> (18.342, -16.149) projected
  line L86 (18.1376, -13.2235) -> (18.1586, -13.2025) projected
  line L87 (18.1586, -13.2025) -> (17.7988, -12.8428) projected
  line L88 (19.5901, 7.3354) -> (18.736, 8.1895) projected
  line L89 (18.9369, 6.2107) -> (19.2338, 6.5076) projected
  line L90 (19.2338, 6.5076) -> (19.2181, 6.5233) projected
  line L91 (18.5282, 7.9817) -> (19.6477, 6.8621) projected
  line L92 (19.6477, 6.8621) -> (19.7962, 7.0106) projected
  line L93 (14.9512, 9.9972) -> (16.5685, 11.6145) projected
  line L94 (16.5685, 11.6145) -> (16.2961, 11.887) projected
  line L95 (16.2961, 11.887) -> (15.0874, 10.6784) projected
  line L96 (14.6491, 11.6896) -> (15.5712, 12.6118) projected
  line L97 (15.5712, 12.6118) -> (15.2988, 12.8843) projected
  line L98 (15.2988, 12.8843) -> (14.2491, 11.8346) projected
  line L99 (14.8569, 10.4478) -> (14.6787, 10.2697) projected
  line L100 (14.6787, 10.2697) -> (14.9512, 9.9972) projected
  line L101 (9.8303, 15.1181) -> (10.1027, 14.8457) projected
  line L102 (10.1027, 14.8457) -> (11.1682, 15.9111) projected
  line L103 (9.708, 18.1187) -> (9.8862, 18.2969) projected
  line L104 (9.8862, 18.2969) -> (9.6137, 18.5694) projected
  line L105 (9.6137, 18.5694) -> (7.9964, 16.952) projected
  line L106 (7.9964, 16.952) -> (8.2689, 16.6796) projected
  line L107 (8.2689, 16.6796) -> (9.4775, 17.8882) projected
  line L108 (9.8495, 16.9712) -> (8.9133, 16.0351) projected
  line L109 (8.9133, 16.0351) -> (9.1858, 15.7626) projected
  line L110 (9.1858, 15.7626) -> (10.2512, 16.828) projected
  line L111 (10.7664, 16.0543) -> (9.8303, 15.1181) projected
  line L112 (18.4037, 13.6419) -> (19.4534, 14.6915) projected
  line L113 (18.8439, 16.0766) -> (19.0238, 16.2565) projected
  line L114 (19.0238, 16.2565) -> (18.7513, 16.5289) projected
  line L115 (18.7513, 16.5289) -> (17.134, 14.9116) projected
  line L116 (17.134, 14.9116) -> (17.4064, 14.6391) projected
  line L117 (17.4064, 14.6391) -> (18.6151, 15.8478) projected
  line L118 (19.0535, 14.8365) -> (18.1313, 13.9143) projected
  line L119 (18.1313, 13.9143) -> (18.4037, 13.6419) projected
  line L120 (17.3261, 16.4137) -> (16.8772, 15.9648) projected
  line L121 (16.6502, 15.7377) -> (16.479, 15.5666) projected
  line L122 (16.479, 15.5666) -> (16.7515, 15.2941) projected
  line L123 (16.7515, 15.2941) -> (17.8571, 16.3997) projected
  line L124 (17.1759, 18.0345) -> (16.8982, 17.7568) projected
  line L125 (16.8982, 17.7568) -> (16.9139, 17.741) projected
  line L126 (17.5951, 16.6826) -> (17.5427, 16.6302) projected
  line L127 (14.2347, 17.8109) -> (16.486, 20.0622) projected
  line L128 (16.486, 20.0622) -> (16.2135, 20.3347) projected
  line L129 (16.2135, 20.3347) -> (13.9622, 18.0834) projected
  line L130 (13.9622, 18.0834) -> (14.2347, 17.8109) projected
  line L131 (13.3789, 20.3609) -> (14.7255, 21.0438) projected
  line L132 (14.7255, 21.0438) -> (14.0443, 19.6955) projected
  line L133 (14.0443, 19.6955) -> (13.3789, 20.3609) projected
  line L134 (11.9676, 20.078) -> (12.2576, 19.788) projected
  line L135 (12.2576, 19.788) -> (13.0558, 20.195) projected
  line L136 (13.0558, 20.195) -> (13.8784, 19.3723) projected
  line L137 (13.8784, 19.3723) -> (13.4714, 18.5742) projected
  line L138 (13.4714, 18.5742) -> (13.7736, 18.272) projected
  line L139 (13.7736, 18.272) -> (15.2023, 21.1538) projected
  line L140 (15.2023, 21.1538) -> (14.8495, 21.5066) projected
  line L141 (14.8495, 21.5066) -> (11.9676, 20.078) projected
  line L142 (-10.6058, 12.9445) -> (-11.5244, 13.8632) projected
  line L143 (-11.7515, 14.0902) -> (-11.9209, 14.2596) projected
  line L144 (-11.9209, 14.2596) -> (-12.1934, 13.9872) projected
  line L145 (-12.1934, 13.9872) -> (-9.9805, 11.7743) projected
  line L146 (-9.9805, 11.7743) -> (-9.708, 12.0467) projected
  line L147 (-9.708, 12.0467) -> (-10.3857, 12.7244) projected
  line L148 (-12.244, 11.3062) -> (-13.1627, 12.2249) projected
  line L149 (-13.3898, 12.4519) -> (-13.5592, 12.6214) projected
  line L150 (-13.5592, 12.6214) -> (-13.8317, 12.3489) projected
  line L151 (-13.8317, 12.3489) -> (-11.6188, 10.136) projected
  line L152 (-11.6188, 10.136) -> (-11.3463, 10.4085) projected
  line L153 (-11.3463, 10.4085) -> (-12.024, 11.0861) projected
  line L154 (-12.6143, 10.3316) -> (-14.2316, 11.9489) projected
  line L155 (-14.2316, 11.9489) -> (-14.5041, 11.6765) projected
  line L156 (-14.5041, 11.6765) -> (-12.8868, 10.0591) projected
  line L157 (-12.8868, 10.0591) -> (-12.6143, 10.3316) projected
  line L158 (-15.8367, 10.8818) -> (-16.1197, 11.1647) projected
  line L159 (-16.1197, 11.1647) -> (-16.4288, 10.8556) projected
  line L160 (-16.4288, 10.8556) -> (-16.1459, 10.5726) projected
  line L161 (-16.1459, 10.5726) -> (-15.8367, 10.8818) projected
  line L162 (-16.3834, 10.363) -> (-16.6384, 10.618) projected
  line L163 (-16.6384, 10.618) -> (-17.9274, 9.3291) projected
  line L164 (-17.9274, 9.3291) -> (-15.7721, 7.1738) projected
  line L165 (-15.7721, 7.1738) -> (-15.4857, 7.4603) projected
  line L166 (-15.4857, 7.4603) -> (-16.5231, 8.4977) projected
  line L167 (-16.5231, 8.4977) -> (-15.5625, 9.4583) projected
  line L168 (-15.5625, 9.4583) -> (-15.8175, 9.7133) projected
  line L169 (-15.8175, 9.7133) -> (-16.7781, 8.7527) projected
  line L170 (-16.7781, 8.7527) -> (-17.3859, 9.3605) projected
  line L171 (-17.3859, 9.3605) -> (-16.3834, 10.363) projected
  line L172 (-7.4589, 22.5842) -> (-9.0762, 24.2015) projected
  line L173 (-9.0762, 24.2015) -> (-9.3487, 23.9291) projected
  line L174 (-9.3487, 23.9291) -> (-7.7313, 22.3117) projected
  line L175 (-7.7313, 22.3117) -> (-7.4589, 22.5842) projected
  line L176 (-9.1111, 20.9319) -> (-10.1608, 21.9816) projected
  line L177 (-11.5458, 21.3721) -> (-11.7257, 21.552) projected
  line L178 (-11.7257, 21.552) -> (-11.9982, 21.2795) projected
  line L179 (-11.9982, 21.2795) -> (-10.3809, 19.6622) projected
  line L180 (-10.3809, 19.6622) -> (-10.1084, 19.9347) projected
  line L181 (-10.1084, 19.9347) -> (-11.317, 21.1433) projected
  line L182 (-10.3058, 21.5817) -> (-9.3836, 20.6595) projected
  line L183 (-9.3836, 20.6595) -> (-9.1111, 20.9319) projected
  line L184 (-11.9109, 20.1093) -> (-12.7649, 19.2552) projected
  line L185 (-10.7861, 19.4561) -> (-11.083, 19.753) projected
  line L186 (-11.083, 19.753) -> (-11.0987, 19.7373) projected
  line L187 (-12.5571, 19.0474) -> (-11.4376, 20.1669) projected
  line L188 (-11.4376, 20.1669) -> (-11.586, 20.3154) projected
  line L189 (-16.3856, 13.6575) -> (-18.6369, 15.9088) projected
  line L190 (-18.6369, 15.9088) -> (-18.9094, 15.6364) projected
  line L191 (-18.9094, 15.6364) -> (-16.658, 13.385) projected
  line L192 (-16.658, 13.385) -> (-16.3856, 13.6575) projected
  line L193 (-18.1653, 13.5719) -> (-17.7165, 13.1231) projected
  line L194 (-17.4894, 12.896) -> (-17.3182, 12.7248) projected
  line L195 (-17.3182, 12.7248) -> (-17.0458, 12.9973) projected
  line L196 (-17.0458, 12.9973) -> (-18.1513, 14.1029) projected
  line L197 (-19.7861, 13.4217) -> (-19.5084, 13.144) projected
  line L198 (-19.5084, 13.144) -> (-19.4927, 13.1597) projected
  line L199 (-18.4343, 13.8409) -> (-18.3819, 13.7885) projected
  line L200 (-20.214, 12.4838) -> (-19.2796, 11.5494) projected
  line L201 (-18.6142, 11.4289) -> (-20.8655, 13.6802) projected
  line L202 (-20.8655, 13.6802) -> (-21.138, 13.4077) projected
  line L203 (-21.138, 13.4077) -> (-20.4394, 12.7091) projected
  line L204 (-19.0508, 11.3206) -> (-18.8867, 11.1564) projected
  line L205 (-18.8867, 11.1564) -> (-18.6142, 11.4289) projected
  line L206 (-21.3598, 10.3775) -> (-20.9109, 9.9286) projected
  line L207 (-20.6839, 9.7015) -> (-20.5127, 9.5304) projected
  line L208 (-20.5127, 9.5304) -> (-20.2402, 9.8028) projected
  line L209 (-20.2402, 9.8028) -> (-21.3458, 10.9084) projected
  line L210 (-22.9806, 10.2272) -> (-22.7029, 9.9495) projected
  line L211 (-22.7029, 9.9495) -> (-22.6872, 9.9653) projected
  line L212 (-21.6288, 10.6464) -> (-21.5764, 10.594) projected
  line L213 (-23.8085, 8.7951) -> (-24.1333, 8.4702) projected
  line L214 (-24.1333, 8.4702) -> (-24.7638, 9.1007) projected
  line L215 (-24.7638, 9.1007) -> (-24.4896, 9.3749) projected
  line L216 (-22.8653, 7.6668) -> (-23.0976, 7.4345) projected
  line L217 (-23.0976, 7.4345) -> (-23.8941, 8.2309) projected
  line L218 (-23.8941, 8.2309) -> (-23.5692, 8.5558) projected
  line L219 (-23.2793, 9.1601) -> (-23.2897, 9.1706) projected
  line L220 (-24.7237, 9.6299) -> (-25.2948, 9.0588) projected
  line L221 (-25.2948, 9.0588) -> (-23.1395, 6.9035) projected
  line L222 (-23.1395, 6.9035) -> (-22.5213, 7.5218) projected
  line L223 (-15.9315, 15.8058) -> (-15.4826, 15.3569) projected
  line L224 (-15.2555, 15.1299) -> (-15.0844, 14.9587) projected
  line L225 (-15.0844, 14.9587) -> (-14.8119, 15.2312) projected
  line L226 (-14.8119, 15.2312) -> (-15.9175, 16.3367) projected
  line L227 (-17.5523, 15.6556) -> (-17.2746, 15.3779) projected
  line L228 (-17.2746, 15.3779) -> (-17.2589, 15.3936) projected
  line L229 (-16.2004, 16.0747) -> (-16.148, 16.0223) projected
  line L230 (-12.5955, 17.4475) -> (-12.3231, 17.72) projected
  line L231 (-12.3231, 17.72) -> (-13.3885, 18.7854) projected
  line L232 (-15.5961, 17.3253) -> (-15.7743, 17.5034) projected
  line L233 (-15.7743, 17.5034) -> (-16.0467, 17.231) projected
  line L234 (-16.0467, 17.231) -> (-14.4294, 15.6137) projected
  line L235 (-14.4294, 15.6137) -> (-14.157, 15.8861) projected
  line L236 (-14.157, 15.8861) -> (-15.3656, 17.0947) projected
  line L237 (-14.4486, 17.4668) -> (-13.5125, 16.5306) projected
  line L238 (-13.5125, 16.5306) -> (-13.24, 16.8031) projected
  line L239 (-13.24, 16.8031) -> (-14.3054, 17.8685) projected
  line L240 (-13.5317, 18.3837) -> (-12.5955, 17.4475) projected
  line L241 (-7.9514, 22.1196) -> (-8.1959, 22.3641) projected
  line L242 (-8.1959, 22.3641) -> (-8.2116, 22.3484) projected
  line L243 (-9.0605, 22.2261) -> (-9.8307, 22.9964) projected
  line L244 (-9.8307, 22.9964) -> (-9.3294, 23.4976) projected
  line L245 (-9.3294, 23.4976) -> (-9.5548, 23.723) projected
  line L246 (-9.5548, 23.723) -> (-10.056, 23.2217) projected
  line L247 (-10.056, 23.2217) -> (-10.5206, 23.6863) projected
  line L248 (-10.5206, 23.6863) -> (-10.7931, 23.4138) projected
  line L249 (-10.7931, 23.4138) -> (-10.3285, 22.9492) projected
  line L250 (-10.3285, 22.9492) -> (-10.5119, 22.7658) projected
  line L251 (-10.5119, 22.7658) -> (-10.2866, 22.5405) projected
  line L252 (-10.2866, 22.5405) -> (-10.1032, 22.7239) projected
  line L253 (-10.1032, 22.7239) -> (-9.2072, 21.8279) projected
  line L254 (-9.326, 24.4897) -> (-9.6089, 24.7726) projected
  line L255 (-9.6089, 24.7726) -> (-9.918, 24.4635) projected
  line L256 (-9.918, 24.4635) -> (-9.6351, 24.1806) projected
  line L257 (-9.6351, 24.1806) -> (-9.326, 24.4897) projected
  line L258 (-13.9696, 8.9763) -> (-15.587, 10.5936) projected
  line L259 (-15.587, 10.5936) -> (-15.8594, 10.3211) projected
  line L260 (-15.8594, 10.3211) -> (-14.2421, 8.7038) projected
  line L261 (-14.2421, 8.7038) -> (-13.9696, 8.9763) projected
  line L262 (-13.292, 9.6539) -> (-15.5433, 11.9053) projected
  line L263 (-15.5433, 11.9053) -> (-15.8158, 11.6328) projected
  line L264 (-15.8158, 11.6328) -> (-13.5644, 9.3815) projected
  line L265 (-13.5644, 9.3815) -> (-13.292, 9.6539) projected
  line L266 (-14.4814, 12.2371) -> (-14.7643, 12.5201) projected
  line L267 (-14.7643, 12.5201) -> (-15.0735, 12.2109) projected
  line L268 (-15.0735, 12.2109) -> (-14.7905, 11.928) projected
  line L269 (-14.7905, 11.928) -> (-14.4814, 12.2371) projected
  line L270 (17.4746, 18.5497) -> (17.7243, 18.7995) projected
  line L271 (16.3341, 19.0545) -> (16.2799, 19.0003) projected
  line L272 (16.2799, 19.0003) -> (16.0965, 19.1837) projected
  line L273 (16.0965, 19.1837) -> (15.8712, 18.9584) projected
  line L274 (15.8712, 18.9584) -> (16.0546, 18.775) projected
  line L275 (16.0546, 18.775) -> (14.6626, 17.383) projected
  line L276 (14.6626, 17.383) -> (14.9351, 17.1105) projected
  line L277 (14.9351, 17.1105) -> (16.3271, 18.5025) projected
  line L278 (16.3271, 18.5025) -> (16.7689, 18.0607) projected
  line L279 (16.7689, 18.0607) -> (16.9943, 18.286) projected
  line L280 (16.9943, 18.286) -> (16.5436, 18.7366) projected
  line L281 (16.5436, 18.7366) -> (16.5978, 18.7907) projected
  line L282 (17.4606, 18.5637) -> (17.4746, 18.5497) projected
  line L283 (6.3546, 18.5938) -> (7.703, 17.2455) projected
  line L284 (7.703, 17.2455) -> (7.958, 17.5005) projected
  line L285 (7.958, 17.5005) -> (6.8961, 18.5624) projected
  line L286 (6.8961, 18.5624) -> (7.696, 19.3623) projected
  line L287 (7.696, 19.3623) -> (8.6863, 18.372) projected
  line L288 (8.6863, 18.372) -> (8.9413, 18.627) projected
  line L289 (8.9413, 18.627) -> (7.951, 19.6173) projected
  line L290 (7.951, 19.6173) -> (8.5413, 20.2076) projected
  line L291 (8.5413, 20.2076) -> (9.6032, 19.1457) projected
  line L292 (9.6032, 19.1457) -> (9.8582, 19.4007) projected
  line L293 (9.8582, 19.4007) -> (8.5099, 20.7491) projected
  line L294 (8.5099, 20.7491) -> (6.3546, 18.5938) projected
  line L295 (12.2336, 14.409) -> (11.7847, 13.9602) projected
  line L296 (11.5576, 13.7331) -> (11.3865, 13.562) projected
  line L297 (11.3865, 13.562) -> (11.6589, 13.2895) projected
  line L298 (11.6589, 13.2895) -> (12.7645, 14.3951) projected
  line L299 (12.0834, 16.0299) -> (11.8056, 15.7521) projected
  line L300 (11.8056, 15.7521) -> (11.8214, 15.7364) projected
  line L301 (12.5025, 14.678) -> (12.4501, 14.6256) projected
  line L302 (13.3112, 11.6372) -> (14.3609, 12.6869) projected
  line L303 (13.7513, 14.072) -> (13.9312, 14.2518) projected
  line L304 (13.9312, 14.2518) -> (13.6588, 14.5243) projected
  line L305 (13.6588, 14.5243) -> (12.0414, 12.907) projected
  line L306 (12.0414, 12.907) -> (12.3139, 12.6345) projected
  line L307 (12.3139, 12.6345) -> (13.5225, 13.8432) projected
  line L308 (13.9609, 12.8319) -> (13.0387, 11.9097) projected
  line L309 (13.0387, 11.9097) -> (13.3112, 11.6372) projected
  line L310 (17.3527, 9.5728) -> (16.4987, 10.4269) projected
  line L311 (16.6995, 8.448) -> (16.9964, 8.7449) projected
  line L312 (16.9964, 8.7449) -> (16.9807, 8.7606) projected
  line L313 (16.2908, 10.219) -> (17.4104, 9.0995) projected
  line L314 (17.4104, 9.0995) -> (17.5588, 9.2479) projected
  line L315 (17.1833, 7.7651) -> (19.4346, 10.0164) projected
  line L316 (19.4346, 10.0164) -> (19.1622, 10.2889) projected
  line L317 (19.1622, 10.2889) -> (16.9109, 8.0376) projected
  line L318 (16.9109, 8.0376) -> (17.1833, 7.7651) projected
  line L319 (13.2961, -17.2686) -> (13.6018, -17.5742) projected
  line L320 (13.6018, -17.5742) -> (13.6175, -17.5585) projected
  line L321 (14.4454, -18.3864) -> (14.4296, -18.4021) projected
  line L322 (14.4296, -18.4021) -> (14.7353, -18.7077) projected
  line L323 (11.312, -19.071) -> (12.9293, -20.6883) projected
  line L324 (12.9293, -20.6883) -> (13.2018, -20.4159) projected
  line L325 (13.2018, -20.4159) -> (11.5845, -18.7985) projected
  line L326 (11.5845, -18.7985) -> (11.312, -19.071) projected
  line L327 (14.7087, -8.5772) -> (14.9637, -8.8322) projected
  line L328 (14.9637, -8.8322) -> (15.926, -7.8699) projected
  line L329 (15.926, -7.8699) -> (17.8263, -9.7701) projected
  line L330 (17.8263, -9.7701) -> (18.1127, -9.4837) projected
  line L331 (18.1127, -9.4837) -> (15.9575, -7.3284) projected
  line L332 (15.9575, -7.3284) -> (14.7087, -8.5772) projected
  line L333 (9.6297, -15.3504) -> (9.1808, -14.9015) projected
  line L334 (8.9537, -14.6745) -> (8.7826, -14.5033) projected
  line L335 (8.7826, -14.5033) -> (8.5101, -14.7758) projected
  line L336 (8.5101, -14.7758) -> (9.6157, -15.8813) projected
  line L337 (11.2505, -15.2002) -> (10.9728, -14.9225) projected
  line L338 (10.9728, -14.9225) -> (10.957, -14.9382) projected
  line L339 (9.8986, -15.6194) -> (9.8462, -15.567) projected
  line L340 (8.5957, -17.3415) -> (8.8786, -17.6244) projected
  line L341 (9.2314, -16.807) -> (9.4725, -17.0481) projected
  line L342 (9.4725, -17.0481) -> (9.7449, -16.7756) projected
  line L343 (9.7449, -16.7756) -> (8.1276, -15.1583) projected
  line L344 (8.1276, -15.1583) -> (7.8551, -15.4307) projected
  line L345 (7.8551, -15.4307) -> (9.0026, -16.5782) projected
  line L346 (8.6097, -17.3275) -> (8.5957, -17.3415) projected
  line L347 (-15.6821, -16.2179) -> (-17.2994, -17.8352) projected
  line L348 (-17.2994, -17.8352) -> (-17.027, -18.1077) projected
  line L349 (-17.027, -18.1077) -> (-15.4097, -16.4904) projected
  line L350 (-15.4097, -16.4904) -> (-15.6821, -16.2179) projected
  line L351 (-16.8873, -15.0407) -> (-17.1318, -15.2853) projected
  line L352 (-17.1318, -15.2853) -> (-17.1161, -15.301) projected
  line L353 (-16.9938, -16.1498) -> (-17.764, -16.92) projected
  line L354 (-17.764, -16.92) -> (-18.2653, -16.4188) projected
  line L355 (-18.2653, -16.4188) -> (-18.4906, -16.6441) projected
  line L356 (-18.4906, -16.6441) -> (-17.9893, -17.1454) projected
  line L357 (-17.9893, -17.1454) -> (-18.4539, -17.6099) projected
  line L358 (-18.4539, -17.6099) -> (-18.1815, -17.8824) projected
  line L359 (-18.1815, -17.8824) -> (-17.7169, -17.4178) projected
  line L360 (-17.7169, -17.4178) -> (-17.5335, -17.6012) projected
  line L361 (-17.5335, -17.6012) -> (-17.3082, -17.3759) projected
  line L362 (-17.3082, -17.3759) -> (-17.4916, -17.1925) projected
  line L363 (-17.4916, -17.1925) -> (-16.5956, -16.2965) projected
  line L364 (-18.3439, -13.5562) -> (-19.9612, -15.1735) projected
  line L365 (-19.9612, -15.1735) -> (-19.6887, -15.4459) projected
  line L366 (-19.6887, -15.4459) -> (-18.0714, -13.8286) projected
  line L367 (-18.0714, -13.8286) -> (-18.3439, -13.5562) projected
  line L368 (-9.0657, -16.0236) -> (-10.0071, -16.965) projected
  line L369 (-10.0071, -16.965) -> (-9.2246, -17.7475) projected
  line L370 (-9.2246, -17.7475) -> (-8.9731, -17.496) projected
  line L371 (-8.9731, -17.496) -> (-9.4727, -16.9965) projected
  line L372 (-9.4727, -16.9965) -> (-8.9155, -16.4393) projected